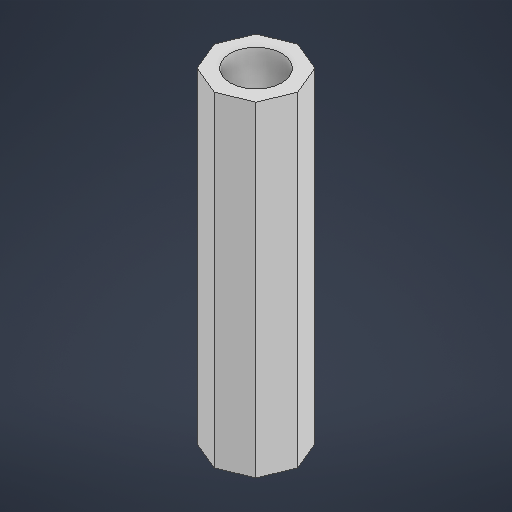
# Autodesk Inventor part: base_telaio_casters
Saved by Autodesk Inventor 2027 (Build 310192060, 192F)
## iProperties
Created: 2026-07-02
Part Number: base_telaio_casters
Material: Generic
Document SubType Name: Modeling
Designer: loren
Density: 1 g/cm^3
Appearance: Default
Author: loren
Autodesk Inventor part; units mm, degrees
ref_plane "YZ Plane" through (0, 0, 0) normal (1, 0, 0) x (0, 1, 0)
ref_plane "XZ Plane" through (0, 0, 0) normal (0, 1, 0) x (-1, 0, 0)
ref_plane "XY Plane" through (0, 0, 0) normal (0, 0, 1) x (1, 0, 0)
sketch "Sketch1" plane through (0, 0, 0) normal (0, 1, 0) x (-1, 0, 0)
  circle A0 centre (0, 0) radius 1.25
  line L0 (0, 0) -> (2.5, 0) construction
  line L1 (1.4352, -1.4352) -> (2.0297, 0)
  line L2 (1.4352, 1.4352) -> (0, 2.0297)
  line L3 (0, 2.0297) -> (-1.4352, 1.4352)
  line L4 (-1.4352, 1.4352) -> (-2.0297, 0)
  line L5 (-2.0297, 0) -> (-1.4352, -1.4352)
  line L6 (-1.4352, -1.4352) -> (0, -2.0297)
  line L7 (0, -2.0297) -> (1.4352, -1.4352)
  line L8 (2.0297, 0) -> (1.4352, 1.4352)
  dimension "d0" = 2.5
  constraints: 18 end point, 2 perpendicular, 1 centre point, 1 coincident, 1 horizontal
  measures "d0" diameter of A0
extrude "Extrusion1" add sketch "Sketch1" along normal blind 15.84
body "Solid1"
